Autodesk Fusion 360 part; units mm, degrees
(part 2 of 2)
sketch "Sketch9" plane through (-29.6, 0, 0) normal (-1, 0, 0) x (0, -1, 0)
  line L0 (-87, -10.02) -> (-84.4, -10.02)
  line L1 (-84.4, -10.02) -> (-84.4, -3.52)
  line L2 (-84.4, -3.52) -> (-87, -3.52)
  line L3 (-87, -3.52) -> (-87, -10.02)
  line L4 (-84.4, -3.52) -> (-84.4, -8.32)
  line L5 (-84.4, -8.32) -> (-83, -8.32)
  line L6 (-84.4, -3.52) -> (-83, -8.32)
  line L7 (-2.6, -3.52) -> (-2.6, -8.32)
  line L8 (-2.6, -8.32) -> (-4, -8.32)
  line L9 (-2.6, -3.52) -> (-4, -8.32)
  dimension "d71" = 4.8
  dimension "d72" = 1.4
  dimension "d73" = 4.8
  dimension "d74" = 1.4
  constraint coincident L1.end L2.start
  constraint perpendicular L2 L4
  constraint perpendicular L4 L5
  constraint vertical L7
  constraint perpendicular L7 L8
  measures "d71" distance of L1.end L4.end
  measures "d72" distance of L4.end L5.end
  measures "d73" distance of L7.start L7.end
  measures "d74" distance of L7.end L8.end
extrude "Extrude16" add sketch "Sketch9" against normal blind 29.2 from surface at -15 contours L1 L4 L5 L6 | L7 L8 L9 bodies 2
sketch "Sketch10" plane through (-29.6, 0, 0) normal (-1, 0, 0) x (0, -1, 0)
  line L0 (-87, -10.02) -> (-84.4, -10.02)
  line L1 (-84.4, -10.02) -> (-84.4, -3.52)
  line L2 (-84.4, -3.52) -> (-87, -3.52)
  line L3 (-87, -3.52) -> (-87, -10.02)
  line L4 (-84.4, -3.52) -> (-81, -10)
  line L5 (-84.4, -3.52) -> (-84.4, -10.02)
  line L6 (-81, -10) -> (-84.4, -10.02)
  line L7 (-2.6, -3.52) -> (-2.6, -10.02)
  line L8 (-2.6, -10.02) -> (-6, -10.02)
  line L9 (-6, -10.02) -> (-2.6, -3.52)
  constraint coincident L1.end L2.start
  constraint coincident L0.end L1.start
  constraint vertical L7
  constraint perpendicular L7 L8
extrude "Extrude17" add sketch "Sketch10" against normal blind 3 contours L1 L4 L5 L6 | L7 L8 L9 bodies 2
extrude "Extrude18" add sketch "Sketch10" along normal blind 3 from surface at -59.2 contours L1 L4 L5 L6 | L7 L8 L9 bodies 2
extrude "Extrude19" add 4 faces at (-8.2683, 83, -18.14) (15.2865, 85, -18.14) (-8.2683, 2, -18.14) (15.2865, 2, -18.14) along direction (0, 0, 1) blind 6 on bodies 2 bodies 2
extrude "Extrude20" add 3 faces at (-16.7972, 31, -19.14) (1.6667, 31, -19.14) (20.1305, 31, -19.14) along direction (0, 0, 1) blind 1.5 on bodies 2 bodies 2
sketch "Sketch11" plane through (23.4639, 0, 0) normal (1, 0, 0) x (0, 1, 0)
  line L0 (6, -17.64) -> (6, -20.64)
  line L1 (6, -20.64) -> (81, -20.64)
  line L2 (81, -20.64) -> (81, -17.64)
  line L3 (81, -17.64) -> (6, -17.64)
  line L4 (81, -17.64) -> (81, -12.64)
  line L5 (81, -17.64) -> (73, -17.64)
  line L6 (73, -17.64) -> (81, -12.64)
  line L7 (6, -17.64) -> (14, -17.64)
  line L8 (6, -17.64) -> (6, -12.64)
  line L9 (6, -12.64) -> (14, -17.64)
  dimension "d87" = 5
  constraint coincident L2.end L3.start
  constraint perpendicular L3 L4
  constraint coincident L3 L5.end
  constraint perpendicular L4 L5
  constraint coincident L0.start L3.end
  constraint coincident L3 L7.end
  constraint perpendicular L0 L7
  constraint perpendicular L7 L8
  measures "d87" distance of L2.end L4.end
extrude "Extrude21" add sketch "Sketch11" along normal blind 3 from surface at -43.5 contours L3 L7 L8 L9 | L3 L4 L5 L6 bodies 2
extrude "Extrude22" add sketch "Sketch11" against normal blind 3 from surface at -3.5 contours L3 L7 L8 L9 | L3 L4 L5 L6 bodies 2
extrude "Extrude23" add sketch "Sketch11" along normal blind 3 from surface at -24.95 contours L3 L7 L8 L9 | L3 L4 L5 L6 bodies 2
